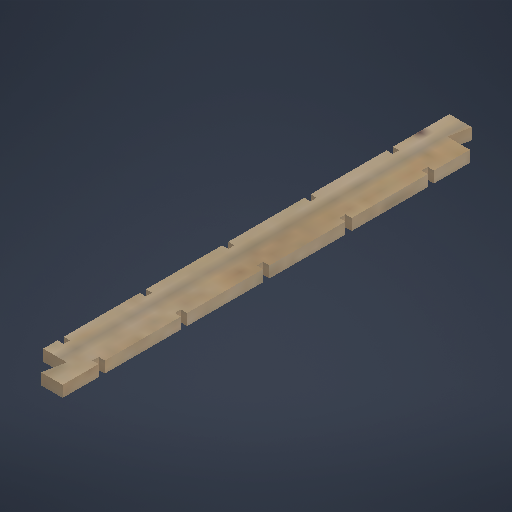
# Autodesk Inventor part: front
Saved by Autodesk Inventor 2026.1 (Build 301233020, 233B)
## iProperties
Created: 2025-09-28
Part Number: front
Material: 木材 (カエデ材)
Document SubType Name: Modeling
Designer: hibik
Density: 0.67 g/cm^3
Appearance: ナチュラル カエデ材 - 光沢 濃い着色
Author: hibik
Autodesk Inventor part; units mm, degrees
ref_plane "YZ Plane" through (0, 0, 0) normal (1, 0, 0) x (0, 1, 0)
ref_plane "XZ Plane" through (0, 0, 0) normal (0, 1, 0) x (-1, 0, 0)
ref_plane "XY Plane" through (0, 0, 0) normal (0, 0, 1) x (1, 0, 0)
sketch "スケッチ1" plane through (0, 0, 0) normal (0, 1, 0) x (-1, 0, 0)
  line L0 (0, 99) -> (20, 99)
  line L1 (20, 99) -> (20, -99)
  line L2 (20, -99) -> (0, -99)
  line L3 (0, -99) -> (0, 99)
  line L4 (20, -99) -> (20, -109)
  line L5 (20, -109) -> (9, -109)
  line L6 (9, -109) -> (11, -99)
  line L7 (10.5, 99) -> (8.5, 88.5)
  line L8 (8.5, 88.5) -> (20, 88.5)
  point P0 (0, 0)
  point P1 (0, 0)
  point P2 (10, -99)
  point P3 (10, 99)
  dimension "d0" = 198
  dimension "d1" = 20
  dimension "d4" = 10
  dimension "d5" = 1
  dimension "d6" = 1
  dimension "d7" = 10.5
  dimension "d8" = 1.5
  dimension "d9" = 0.5
  constraints: 18 end point, 3 midpoint, 3 perpendicular, 3 point on line, 2 parallel, 1 coincident, 1 horizontal, 1 vertical
  measures "d0" distance of L0.end L1.end
  measures "d1" distance of L0.start L0.end
  measures "d4" distance of L1.end L4.end
  measures "d5" distance of point (10, -99) L6.end
  measures "d6" horizontal distance of point (10, -99) L5.end
  measures "d7" distance between parallel lines of L0 L8
  measures "d8" horizontal distance of point (10, 99) L7.end
  measures "d9" distance of point (10, 99) L7.start
extrude "押し出し1" add sketch "スケッチ1" along normal blind 5.5 contours L0 L7 L8 L1 L2 L3 | L2 L4 L5 L6
sketch "スケッチ2" plane through (0, 5.5, 0) normal (0, 1, 0) x (1, 0, 0)
  line L0 (-20, 109) -> (-20, -88.5) projected
  line L1 (-20, -1.5) -> (-17, -1.5)
  line L2 (-17, -1.5) -> (-17, 1.5)
  line L3 (-17, 1.5) -> (-20, 1.5)
  line L4 (-20, 1.5) -> (-20, -1.5)
  line L5 (0, -99) -> (0, 99) projected
  line L6 (0, -1.5) -> (-3, -1.5)
  line L7 (-3, -1.5) -> (-3, 1.5)
  line L8 (-3, 1.5) -> (0, 1.5)
  line L9 (0, 1.5) -> (0, -1.5)
  point P0 (0, 0)
  point P1 (-17, 0)
  point P2 (0, 0)
  point P3 (0, 1.5)
  dimension "d10" = 3
  dimension "d11" = 3
  constraints: 16 end point, 4 parallel, 4 point on line, 2 horizontal, 2 midpoint, 2 perpendicular, 1 collinear, 1 horizontal alignment
  measures "d10" distance of L1.start L1.end
  measures "d11" distance of L1.end L2.end
extrude "押し出し2" cut sketch "スケッチ2" against normal through all
pattern_linear "矩形状パターン1" count 3 spacing 40 along (0, 0, -1) count 3 spacing 40 along (0, 0, 1) of "押し出し2"
